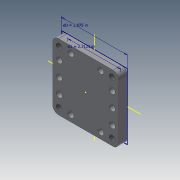
# Autodesk Inventor part: Standard
Saved by Autodesk Inventor 2020.3 (Build 243373000, 373)
## iProperties
RuleStatus: InUse
AfterDocSave0: file://Part Number Cleaner
Created: 2022-10-11
Material: Generic
Catalog Web Link: https://www.janelia.org/
Vendor: HHMI: JRC - jET
Document SubType Name: Modeling
Designer: arnoldj
Density: 1 g/cm^3
Appearance: Default
DESIGN DEPARTMENT: HHMI: JRC - jET
ALTERED ITEM PART NUMBER: N/A
ALTERED ITEM VENDOR: N/A
ALTERED ITEM DESCRIPTION: N/A
Title: Standard
Author: arnoldj
Revision Number: 0
Autodesk Inventor part; units mm, degrees
ref_plane "YZ Plane" through (0, 0, 0) normal (1, 0, 0) x (0, 1, 0)
ref_plane "XZ Plane" through (0, 0, 0) normal (0, 1, 0) x (-1, 0, 0)
ref_plane "XY Plane" through (0, 0, 0) normal (0, 0, 1) x (1, 0, 0)
sketch "Sketch1" plane through (0, 0, 0) normal (0, 0, 1) x (1, 0, 0)
  line L0 (0, 51.1175) -> (0, -51.1175) projected
  line L1 (-51.1175, 0) -> (51.1175, 0) projected
  line L2 (36.5125, -36.5125) -> (-36.5125, -36.5125)
  line L3 (-36.5125, -36.5125) -> (-36.5125, 36.5125)
  line L4 (-36.5125, 36.5125) -> (36.5125, 36.5125)
  line L5 (36.5125, 36.5125) -> (36.5125, -36.5125)
  line L6 (36.5125, -36.5125) -> (-36.5125, 36.5125) construction
  line L7 (-36.5125, -36.5125) -> (36.5125, 36.5125) construction
  line L8 (29.3688, -29.3688) -> (-29.3688, -29.3688) construction
  line L9 (-29.3688, -29.3688) -> (-29.3688, 29.3687) construction
  line L10 (-29.3688, 29.3687) -> (29.3688, 29.3687) construction
  line L11 (29.3688, 29.3687) -> (29.3688, -29.3688) construction
  line L12 (29.3688, -29.3688) -> (-29.3688, 29.3687) construction
  line L13 (-29.3688, -29.3688) -> (29.3688, 29.3687) construction
  point P0 (0, 0)
  dimension "d0" = 73.025
  dimension "d1" = 58.7375
  constraints: 24 end point, 4 coincident, 4 midpoint, 4 parallel, 4 perpendicular, 2 horizontal
  measures "d0" distance of L3.end L4.end
  measures "d1" distance of L9.end L10.end
extrude "Extrusion1" add sketch "Sketch1" along normal blind 9.525
hole "Hole1" at (-29.3688, 29.3687, 0) at (29.3688, 29.3687, 0) at (29.3688, -29.3688, 0) at (-29.3688, -29.3688, 0) direction (0, 0, 1) diameter 6.647 end through all thread size "M8x1.25" class "6H" standard "ANSI Metric M Profile"
sketch "Sketch2" plane through (0, 0, 0) normal (0, 0, -1) x (-1, 0, 0)
  line L0 (-36.5125, 36.5125) -> (36.5125, 36.5125) projected
  line L1 (-29.3688, 29.3687) -> (-29.3688, -29.3688) construction
  line L2 (29.3688, -29.3688) -> (29.3688, 29.3687) construction
  line L3 (29.3688, 29.3687) -> (-29.3688, 29.3687) construction
  line L4 (-29.3688, -29.3688) -> (29.3688, -29.3688) construction
  line L5 (16.5125, -29.3687) -> (-16.5125, -29.3687) construction
  line L6 (-16.5125, -29.3687) -> (-16.5125, 29.3687) construction
  line L7 (-16.5125, 29.3687) -> (16.5125, 29.3687) construction
  line L8 (16.5125, 29.3687) -> (16.5125, -29.3687) construction
  line L9 (16.5125, -29.3687) -> (-16.5125, 29.3687) construction
  line L10 (-16.5125, -29.3687) -> (16.5125, 29.3687) construction
  line L11 (-36.5125, -36.5125) -> (-36.5125, 36.5125) construction
  line L12 (29.3688, -16.5125) -> (-29.3688, -16.5125) construction
  line L13 (-29.3688, -16.5125) -> (-29.3688, 16.5125) construction
  line L14 (-29.3688, 16.5125) -> (29.3688, 16.5125) construction
  line L15 (29.3688, 16.5125) -> (29.3688, -16.5125) construction
  line L16 (29.3688, -16.5125) -> (-29.3688, 16.5125) construction
  line L17 (-29.3688, -16.5125) -> (29.3688, 16.5125) construction
  point P0 (0, 0)
  point P1 (-29.3688, 0)
  point P2 (29.3688, 0)
  point P3 (0, 29.3687)
  point P4 (0, -29.3688)
  dimension "d12" = 20
  dimension "d21" = 20
  constraints: 24 end point, 8 coincident, 8 midpoint, 4 parallel, 2 horizontal, 2 perpendicular, 2 point on line
  measures "d12" distance between parallel lines of L6 L11
  measures "d21" distance between parallel lines of L14 L0
hole "Hole2" at (-16.5125, 29.3687, 0) at (16.5125, -29.3687, 0) at (29.3688, 0, 0) at (-29.3688, 0, 0) at (16.5125, 29.3687, 0) at (-16.5125, -29.3687, 0) at (29.3688, 16.5125, 0) at (29.3688, -16.5125, 0) at (-29.3688, -16.5125, 0) at (-29.3688, 16.5125, 0) direction (0, 0, 1) diameter 6.604 end through all countersink diameter 12.5984 countersink angle 90 clearance for "Flat Head Machine Screw" size "M6" standard "Ansi Metric M Profile"
fillet "Fillet1" radius 6.35 4 edges at (-36.5125, -36.5125, 4.7625) (-36.5125, 36.5125, 4.7625) (36.5125, -36.5125, 4.7625) (36.5125, 36.5125, 4.7625)
sketch "Sketch3" plane through (0, 0, 9.525) normal (0, 0, 1) x (1, 0, 0)
  point P0 (0, 0)
body "Solid1"
